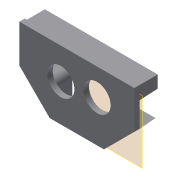
# Autodesk Inventor part: 30_Baseplate_Connector_Clamp
Saved by Autodesk Inventor 2019 (Build 230136000, 136)
## iProperties
Created: 2020-01-13
Part Number: 30_Baseplate_Connector_Clamp
Material: Generic
Document SubType Name: Modeling
Designer: diederichbenedict
Density: 1 g/cm^3
Appearance: Default
Author: diederichbenedict
Autodesk Inventor part; units mm, degrees
ref_plane "YZ Plane" through (0, 0, 0) normal (1, 0, 0) x (0, 1, 0)
ref_plane "XZ Plane" through (0, 0, 0) normal (0, 1, 0) x (-1, 0, 0)
ref_plane "Work Plane1" through (50, -100, 0) normal (0, 0, 1) x (1, 0, 0)
sketch "Sketch1" plane through (50, -100, 0) normal (0, 0, 1) x (1, 0, 0)
  line L0 (-9.1, 25) -> (-9.1, 17.5) construction
  line L1 (-9.1, 25) -> (-25, 25) construction
  line L2 (-25, 25) -> (-25, 9.1) construction
  line L3 (-17.5, 9.1) -> (-25, 9.1) construction
  line L4 (-17.5, 9.1) -> (-17.5, 15.5) construction
  arc A0 (-15.5, 17.5) -> (-17.5, 15.5) centre (-15.5, 15.5) ccw construction
  line L5 (-15.5, 17.5) -> (-9.1, 17.5) construction
  circle A1 centre (-20, 20) radius 2.2989 construction
  line L6 (-40.9, 17.5) -> (-40.9, 25)
  line L7 (-40.9, 17.5) -> (-34.5, 17.5) construction
  arc A2 (-32.5, 15.5) -> (-34.5, 17.5) centre (-34.5, 15.5) ccw construction
  line L8 (-32.5, 15.5) -> (-32.5, 9.1) construction
  line L9 (-25, 9.1) -> (-32.5, 9.1)
  line L10 (-25, 9.1) -> (-25, 25) construction
  line L11 (-25, 25) -> (-40.9, 25) construction
  circle A3 centre (-30, 20) radius 2.2989 construction
  line L12 (-40.9, 25) -> (-40.9, 32.5) construction
  line L13 (-40.9, 25) -> (-25, 25)
  line L14 (-25, 25) -> (-25, 40.9) construction
  line L15 (-32.5, 40.9) -> (-25, 40.9) construction
  line L16 (-32.5, 40.9) -> (-32.5, 34.5) construction
  arc A4 (-34.5, 32.5) -> (-32.5, 34.5) centre (-34.5, 34.5) ccw construction
  line L17 (-34.5, 32.5) -> (-40.9, 32.5) construction
  circle A5 centre (-30, 30) radius 2.2989 construction
  circle A6 centre (-20, 30) radius 2.2989 construction
  line L18 (-25, 40.9) -> (-17.5, 40.9) construction
  line L19 (-25, 40.9) -> (-25, 25) construction
  line L20 (-25, 25) -> (-9.1, 25) construction
  line L21 (-9.1, 32.5) -> (-9.1, 25) construction
  line L22 (-9.1, 32.5) -> (-15.5, 32.5) construction
  arc A7 (-17.5, 34.5) -> (-15.5, 32.5) centre (-15.5, 34.5) ccw construction
  line L23 (-17.5, 34.5) -> (-17.5, 40.9) construction
  line L24 (-25, 9.1) -> (-32.5, 9.1)
  line L25 (-40.9, 17.5) -> (-32.5, 9.1)
  line L26 (-40.9, 17.5) -> (-40.9, 25)
  line L27 (-25, 25) -> (-40.9, 25)
  line L28 (-25, 9.1) -> (-25, 25)
  arc A8 (-32.5755, 19.3934) -> (-26.2755, 19.3934) centre (-29.4255, 19.3934) ccw projected
  circle A9 centre (-29.4255, 19.3934) radius 3.75
  line L29 (-40.9, 17.5) -> (-40.9, 25) projected
  line L30 (-25, 9.1) -> (-32.5, 9.1) projected
  line L31 (-40.9, 25) -> (-25, 25) projected
  point P0 (-50, 100)
  dimension "d0" = 7.5
  constraints: 16 end point, 3 collinear, 1 centre point, 1 coincident
  measures "d0" diameter of A9
extrude "Extrusion1" add sketch "Sketch1" along normal blind 1.5
sketch "Sketch2" plane through (50, -100, 0) normal (0, 0, -1) x (-1, 0, 0)
  circle A0 centre (29.4255, 19.3934) radius 3.75 projected
  line L0 (25, 25) -> (40.9, 25) projected
  line L1 (25, 9.1) -> (25, 25) projected
  line L2 (32.5, 9.1) -> (25, 9.1) projected
  line L3 (40.9, 17.5) -> (32.5, 9.1) projected
  line L4 (40.9, 25) -> (40.9, 17.5) projected
  line L5 (32.5, -15.5) -> (32.5, 15.5) projected
  arc A1 (34.5, 17.5) -> (32.5, 15.5) centre (34.5, 15.5) ccw projected
  line L6 (34.5, 17.5) -> (65.5, 17.5) projected
  line L7 (65.9987, 17.7) -> (34.5, 17.7)
  arc A2 (34.5, 17.7) -> (32.3, 15.5) centre (34.5, 15.5) ccw
  line L8 (32.3, 15.5) -> (32.3, -15.5)
  line L9 (40.9, 17.5) -> (32.5, 9.1) projected
  point P0 (50, 100)
  point P1 (41.1, 17.7)
  point P2 (32.3, 8.9)
  dimension "d9" = 0.2
  constraints: 4 end point, 4 point on line, 2 point on circle, 1 centre point, 2 other
  measures "d9" distance between parallel lines of L6 L7
extrude "Extrusion2" add sketch "Sketch2" along normal blind 5 draft -3 contours L3 L5 A1 L6
pattern_circular "Circular Pattern1" count 2 over 90 about axis through (25, -75, 0) along (0, 0, 1) of "Extrusion1", "Extrusion2"
sketch "Sketch3" plane through (50, -100, 1.5) normal (0, 0, 1) x (1, 0, 0)
  circle A0 centre (-19.3934, 20.5745) radius 3.75 projected
  circle A1 centre (-29.4255, 19.3934) radius 3.75 projected
  line L0 (-9.1, 25) -> (-40.9, 25) projected
  line L1 (-40.9, 25) -> (-40.9, 17.5) projected
  line L2 (-40.9, 17.5) -> (-32.5, 9.1) projected
  line L3 (-32.5, 9.1) -> (-17.5, 9.1) projected
  line L4 (-17.5, 9.1) -> (-9.1, 17.5) projected
  line L5 (-9.1, 17.5) -> (-9.1, 25) projected
  line L6 (-40.9, 25) -> (-9.1, 25)
  line L7 (-9.1, 25) -> (-9.1, 28)
  line L8 (-9.1, 28) -> (-40.9, 28)
  line L9 (-40.9, 28) -> (-40.9, 25)
  point P0 (-50, 100)
  dimension "d10" = 3
  constraints: 8 end point, 2 parallel, 1 horizontal, 1 perpendicular
  measures "d10" distance of L7.end L6.end
ref_plane "Work Plane2" through (25.5745, -91.5066, 0) normal (0, 0, 1) x (1, 0, 0)
extrude "Extrusion3" add sketch "Sketch3" against normal up to surface (1.5 mm away) contours L0 L9 L8 L7
sketch "Sketch4" plane through (40.9, -82.5, 1.5) normal (1, 0, 0) x (0, 0, -1)
  line L0 (1.5, 6.8934) -> (9.5, 6.8934) construction
  line L1 (6.5, -7.7674) -> (6.5, -0.262) projected
  line L2 (1.5, 0) -> (1.5, 10.5) construction
  line L3 (1.5, 10.5) -> (6.5, 10.5) construction
  line L4 (0, 10.5) -> (1.5, 10.5) projected
  line L5 (1.5, 10.5) -> (6.5, 10.5)
  line L6 (1.5, 10.5) -> (1.5, 6.6716)
  line L7 (6.5, 10.5) -> (6.5, 7.1108) construction
  line L8 (6.5, 7.1108) -> (1.5, 6.8487)
  line L9 (1.5, 6.8487) -> (1.5, 10.5)
  line L10 (6.5, 10.5) -> (6.5, 7.1108)
  point P0 (1.5, 82.5)
  dimension "d16" = 93
  constraints: 16 end point, 2 collinear, 2 horizontal, 2 point on line, 1 parallel, 1 vertical, 2 other
  measures "d16" angle of L7 L8
extrude "Extrusion4" add sketch "Sketch4" against normal up to surface (31.2255 mm away)
body "Solid1"
